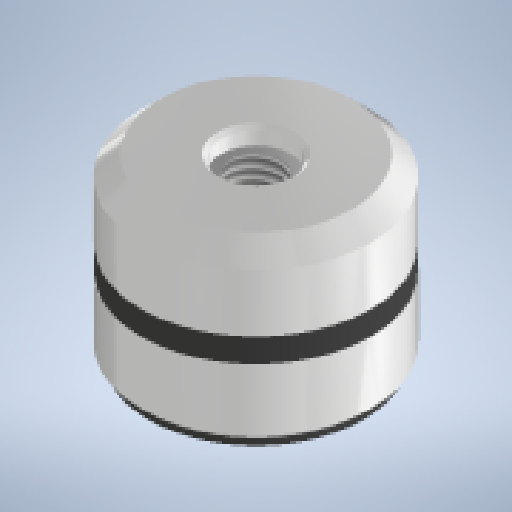
# Autodesk Inventor part: Levelling Foot R2
Saved by Autodesk Inventor 2024 (Build 280153000, 153)
## iProperties
Created: 2024-10-28
Part Number: Levelling Foot R2
Material: ABS Plastic
Document SubType Name: Modeling
Designer: Ishaan
Density: 1.06 g/cm^3
Appearance: Smooth - White
Author: Ishaan
Autodesk Inventor part; units mm, degrees
ref_plane "YZ Plane" through (0, 0, 0) normal (1, 0, 0) x (0, 1, 0)
ref_plane "XZ Plane" through (0, 0, 0) normal (0, 1, 0) x (-1, 0, 0)
sketch "Sketch1" plane through (0, 0, 0) normal (0, 0, 1) x (1, 0, 0)
  line L0 (0, 0) -> (-15, 0)
  line L1 (-15, 0) -> (-15, -10)
  line L2 (-15, -10) -> (-6, -12.4115)
  line L3 (-6, -12.4115) -> (-6, -18)
  line L4 (-6, -18) -> (0, -18)
  line L5 (0, -18) -> (0, 0)
  line L6 (-15, -10) -> (-15, -11.5529)
  line L7 (-15, -11.5529) -> (-15, -13.1058)
  line L8 (-14, -23) -> (0, -23)
  line L9 (0, -23) -> (0, -18)
  line L10 (-15, -13.1058) -> (-9, -14.7135)
  line L11 (-9, -14.7135) -> (-9, -18)
  line L12 (-9, -18) -> (-12, -18)
  line L13 (-12, -22) -> (-15, -22)
  line L14 (-15, -13.1058) -> (-15, -22)
  line L15 (-12, -18) -> (-12, -22)
  line L16 (-14, -23) -> (-14, -22)
  line L17 (-14.6118, -10.104) -> (-15.3882, -13.0018) construction
  line L18 (0, -27.6) -> (0, 4.6) projected
  dimension "d0" = 15
  dimension "d1" = 10
  dimension "d2" = 105
  dimension "d3" = 18
  dimension "d4" = 6
  dimension "d6" = 3
  dimension "d8" = 3
  dimension "d9" = 5
  dimension "d10" = 1
  dimension "d11" = 2
  dimension "d12" = 1
  dimension "d13" = 15
  constraints: 37 end point, 6 perpendicular, 4 vertical, 3 point on line, 2 horizontal, 2 parallel, 1 collinear, 1 midpoint
  measures "d0" distance of L0.start L0.end
  measures "d1" distance of L0.end L1.end
  measures "d2" angle of L1 L2
  measures "d3" distance of L4.end L0.start
  measures "d4" distance between parallel lines of L5 L3
  measures "d6" distance between parallel lines of L2 L10
  measures "d8" distance between parallel lines of L3 L11
  measures "d9" distance between parallel lines of L12 L8
  measures "d10" distance between parallel lines of L14 L16
  measures "d11" distance between parallel lines of L16 L15
  measures "d12" distance between parallel lines of L8 L13
  measures "d13" distance between parallel lines of L9 L14
revolve "Revolution1" add sketch "Sketch1" angle 360 about axis through (0, -10, 0) along (0, 1, 0) contours L5 L4 L3 L2 L1 L0
revolve "Revolution2" add sketch "Sketch1" angle 360 about axis through (0, -10, 0) along (0, 1, 0) separate body contours L9 L8 L16 L13 L15 L12 L11 L10 L7 L6 L2 L3 L4
revolve "Revolution3" add sketch "Sketch1" angle 360 about axis through (0, -10, 0) along (0, 1, 0) separate body contours L10 L11 L12 L15 L13 L14
sketch "Sketch2" plane through (0, 0, 0) normal (0, 1, 0) x (1, 0, 0)
  circle A0 centre (0, 0) radius 15 projected
  constraints: 1 coincident
hole "Hole1" at (0, 0, 0) direction (0, -1, 0) diameter 9 end through all bodies 1 2 3
chamfer "Chamfer1" distance 2 angle 45 1 edges at (0, -23, -4.5)
ref_plane "Work Plane1" through (0, -5.5, 0) normal (0, 1, 0) x (1, 0, 0)
sketch "Sketch3" plane through (0, -5.5, 0) normal (0, 1, 0) x (1, 0, 0)
  circle A0 centre (0, 0) radius 12
  circle A1 centre (12, 0) radius 4
  circle A2 centre (6, 10.3923) radius 4
  circle A3 centre (-6, 10.3923) radius 4
  circle A4 centre (-12, 0) radius 4
  circle A5 centre (-6, -10.3923) radius 4
  circle A6 centre (6, -10.3923) radius 4
  point P0 (2.251, -11.787)
  point P1 (9.0823, -7.8429)
  point P2 (11.3333, -3.9441)
  point P3 (11.3333, 3.9441)
  point P4 (9.0823, 7.8429)
  point P5 (2.251, 11.787)
  point P6 (-2.251, 11.787)
  point P7 (-9.0823, 7.8429)
  point P8 (-11.3333, 3.9441)
  point P9 (-11.3333, -3.9441)
  point P10 (-9.0823, -7.8429)
  point P11 (-2.251, -11.787)
  dimension "d40" = 24
  dimension "d41" = 8
  dimension "d44" = 360
  constraints: 6 centre point, 1 coincident, 1 horizontal alignment, 16 other
  measures "d41" diameter of A1
extrude "Extrusion1" cut sketch "Sketch3" along normal mid plane 6.6 contours A1 A0 A6 A5 A4 A3 A2 bodies 1
fillet "Fillet3" radius 1 12 edges at (-11.3333, -5.5, 3.9441) (-9.0823, -5.5, 7.8429) (-11.3333, -5.5, -3.9441) (-9.0823, -5.5, -7.8429) (-2.251, -5.5, -11.787) (2.251, -5.5, -11.787) (9.0823, -5.5, -7.8429) (11.3333, -5.5, -3.9441) (11.3333, -5.5, 3.9441) (9.0823, -5.5, 7.8429) (2.251, -5.5, 11.787) (-2.251, -5.5, 11.787)
sketch "Sketch4" plane through (0, -2.2, 0) normal (0, -1, 0) x (1, 0, 0)
  point P0 (0, 0)
sketch "Sketch5" plane through (0, -5.5, 0) normal (0, 1, 0) x (1, 0, 0)
  arc A0 (-9.784, -6.948) -> (-8.3749, -7.1736) centre (-8.9686, -6.369) ccw projected
  arc A1 (-2.0251, -10.8397) -> (-8.3749, -7.1736) centre (-6, -10.3923) ccw projected
  arc A2 (-2.0251, -10.8397) -> (-1.1251, -11.9471) centre (-1.0314, -10.9515) ccw projected
  arc A3 (-1.1251, -11.9471) -> (1.1251, -11.9471) centre (0, 0) ccw projected
  arc A4 (1.1251, -11.9471) -> (2.0251, -10.8397) centre (1.0314, -10.9515) ccw projected
  arc A5 (8.3749, -7.1736) -> (2.0251, -10.8397) centre (6, -10.3923) ccw projected
  arc A6 (8.3749, -7.1736) -> (9.784, -6.948) centre (8.9686, -6.369) ccw projected
  arc A7 (9.784, -6.948) -> (10.9091, -4.9992) centre (0, 0) ccw projected
  arc A8 (10.9091, -4.9992) -> (10.4, -3.6661) centre (10, -4.5826) ccw projected
  arc A9 (10.4, 3.6661) -> (10.4, -3.6661) centre (12, 0) ccw projected
  arc A10 (10.4, 3.6661) -> (10.9091, 4.9992) centre (10, 4.5826) ccw projected
  arc A11 (10.9091, 4.9992) -> (9.784, 6.948) centre (0, 0) ccw projected
  arc A12 (9.784, 6.948) -> (8.3749, 7.1736) centre (8.9686, 6.369) ccw projected
  arc A13 (2.0251, 10.8397) -> (8.3749, 7.1736) centre (6, 10.3923) ccw projected
  arc A14 (2.0251, 10.8397) -> (1.1251, 11.9471) centre (1.0314, 10.9515) ccw projected
  arc A15 (1.1251, 11.9471) -> (-1.1251, 11.9471) centre (0, 0) ccw projected
  arc A16 (-1.1251, 11.9471) -> (-2.0251, 10.8397) centre (-1.0314, 10.9515) ccw projected
  arc A17 (-8.3749, 7.1736) -> (-2.0251, 10.8397) centre (-6, 10.3923) ccw projected
  arc A18 (-8.3749, 7.1736) -> (-9.784, 6.948) centre (-8.9686, 6.369) ccw projected
  arc A19 (-9.784, 6.948) -> (-10.9091, 4.9992) centre (0, 0) ccw projected
  arc A20 (-10.9091, 4.9992) -> (-10.4, 3.6661) centre (-10, 4.5826) ccw projected
  arc A21 (-10.4, -3.6661) -> (-10.4, 3.6661) centre (-12, 0) ccw projected
  arc A22 (-10.4, -3.6661) -> (-10.9091, -4.9992) centre (-10, -4.5826) ccw projected
  arc A23 (-10.9091, -4.9992) -> (-9.784, -6.948) centre (0, 0) ccw projected
  circle A24 centre (0, 0) radius 15 projected
  arc A25 (-1.097, 11.6485) -> (-1.727, 10.8732) centre (-1.0314, 10.9515) ccw
  arc A26 (1.097, 11.6485) -> (-1.097, 11.6485) centre (0, 0) ccw
  arc A27 (1.727, 10.8732) -> (1.097, 11.6485) centre (1.0314, 10.9515) ccw
  arc A28 (1.727, 10.8732) -> (8.553, 6.9322) centre (6, 10.3923) ccw
  arc A29 (9.5394, 6.7743) -> (8.553, 6.9322) centre (8.9686, 6.369) ccw
  arc A30 (10.6364, 4.8742) -> (9.5394, 6.7743) centre (0, 0) ccw
  arc A31 (10.28, 3.941) -> (10.6364, 4.8742) centre (10, 4.5826) ccw
  arc A32 (10.28, 3.941) -> (10.28, -3.941) centre (12, 0) ccw
  arc A33 (10.6364, -4.8742) -> (10.28, -3.941) centre (10, -4.5826) ccw
  arc A34 (9.5394, -6.7743) -> (10.6364, -4.8742) centre (0, 0) ccw
  arc A35 (8.553, -6.9322) -> (9.5394, -6.7743) centre (8.9686, -6.369) ccw
  arc A36 (8.553, -6.9322) -> (1.727, -10.8732) centre (6, -10.3923) ccw
  arc A37 (1.097, -11.6485) -> (1.727, -10.8732) centre (1.0314, -10.9515) ccw
  arc A38 (-1.097, -11.6485) -> (1.097, -11.6485) centre (0, 0) ccw
  arc A39 (-1.727, -10.8732) -> (-1.097, -11.6485) centre (-1.0314, -10.9515) ccw
  arc A40 (-1.727, -10.8732) -> (-8.553, -6.9322) centre (-6, -10.3923) ccw
  arc A41 (-9.5394, -6.7743) -> (-8.553, -6.9322) centre (-8.9686, -6.369) ccw
  arc A42 (-10.6364, -4.8742) -> (-9.5394, -6.7743) centre (0, 0) ccw
  arc A43 (-10.28, -3.941) -> (-10.6364, -4.8742) centre (-10, -4.5826) ccw
  arc A44 (-10.28, -3.941) -> (-10.28, 3.941) centre (-12, 0) ccw
  arc A45 (-10.6364, 4.8742) -> (-10.28, 3.941) centre (-10, 4.5826) ccw
  arc A46 (-9.5394, 6.7743) -> (-10.6364, 4.8742) centre (0, 0) ccw
  arc A47 (-8.553, 6.9322) -> (-9.5394, 6.7743) centre (-8.9686, 6.369) ccw
  arc A48 (-8.553, 6.9322) -> (-1.727, 10.8732) centre (-6, 10.3923) ccw
  dimension "d49" = 0.3
  constraints: 48 point on circle, 24 centre point, 23 other
  measures "d49" radial gap between concentric circles of A17 A48
extrude "Extrusion2" add sketch "Sketch5" along normal mid plane 6.35 separate body contours A26 A27 A28 A29 A30 A31 A32 A33 A34 A35 A36 A37 A38 A39 A40 A41 A42 A43 A44 A45 A46 A47 A48 A25
sketch "Sketch6" plane through (0, -2.325, 0) normal (0, 1, 0) x (1, 0, 0)
  arc A0 (-1.1251, -11.9471) -> (1.1251, -11.9471) centre (0, 0) ccw projected
  constraints: 1 coincident
hole "Hole2" at (0, -2.325, 0) direction (0, -1, 0) diameter 6.647 end through all bodies 4 thread size "M8x1.25" class "6H" standard "ANSI Metric M Profile"
chamfer "Chamfer2" distance 0.5 angle 45 1 edges at (0, 0, -4.5)
chamfer "Chamfer3" distance 0.75 angle 45 1 edges at (15, -22, 0)
chamfer "Chamfer4" distance 2.5 angle 45 1 edges at (15, 0, 0)
equation "\"d8\" = d6"
equation "\"d13\" = d0"
